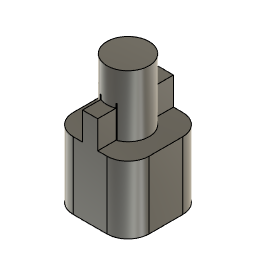
twomes-p1-gateway-button (Autodesk Fusion 360 design; units mm, degrees)
Autodesk Fusion 360 part; units mm, degrees
sketch "Sketch1" plane through (0, 0, 0) normal (0, 1, 0) x (1, 0, 0) in component "RectangleBaseCap"
  line L0 (8.6959, 0, -1.1385) -> (17.6959, 0, -1.1385)
  line L1 (17.6959, 0, -1.1385) -> (17.6959, 0, 7.8615)
  line L2 (17.6959, 0, 7.8615) -> (8.6959, 0, 7.8615)
  line L3 (8.6959, 0, 7.8615) -> (8.6959, 0, -1.1385)
  dimension "d21" = 9
  dimension "d22" = 9
extrude "Extrude1" add sketch "Sketch1" against normal blind 7 contours L0 L1 L2 L3 in plane through (0, 0, 0) normal (0, 0, -1) in component "RectangleBaseCap"
sketch "Sketch2" plane through (0, 0, 7) normal (0, 0, 1) x (-1, 0, 0) in component "RectangleBaseCap"
  line L0 (-8.6959, -7.8615) -> (-8.6959, 1.1385)
  line L1 (-8.6959, 1.1385) -> (-17.6959, 1.1385)
  line L2 (-17.6959, 1.1385) -> (-17.6959, -7.8615)
  line L3 (-17.6959, -7.8615) -> (-8.6959, -7.8615)
  circle A0 centre (-13.1959, -3.3615) radius 2.5
  dimension "d25" = 5
  measures "d25" diameter of A0
extrude "Extrude2" add sketch "Sketch2" along normal blind 5 contours A0 in component "RectangleBaseCap"
move_body "Move1" [no effect]
extrude "Extrude3" add 1 faces at (11.6959, 1.8615, 0) along direction (0, 0, -1) blind 4 in component "RectangleBaseCap"
sketch "Sketch3" plane through (0, 0, -4) normal (0, 0, -1) x (1, 0, 0) in component "RectangleBaseCap"
  line L0 (8.6959, 1.1385) -> (8.6959, -7.8615)
  line L1 (8.6959, -7.8615) -> (17.6959, -7.8615)
  line L2 (17.6959, -7.8615) -> (17.6959, 1.1385)
  line L3 (17.6959, 1.1385) -> (8.6959, 1.1385)
  line L4 (9.6959, -6.8615) -> (16.6959, -6.8615)
  line L5 (16.6959, -6.8615) -> (16.6959, 0.1385)
  line L6 (16.6959, 0.1385) -> (9.6959, 0.1385)
  line L7 (9.6959, 0.1385) -> (9.6959, -6.8615)
  line L8 (8.6959, -3.3615) -> (9.6959, -3.3615) construction
  line L9 (13.1959, -7.8615) -> (13.1959, -6.8615) construction
  dimension "d30" = 7
  dimension "d31" = 7
  constraint horizontal L4
  constraint vertical L5
  constraint horizontal L6
  constraint vertical L7
  constraint midpoint L0 L8.start
  constraint midpoint L7 L8.end
  constraint perpendicular L0 L8
  constraint midpoint L1 L9.start
  constraint midpoint L4 L9.end
  constraint perpendicular L1 L9
  measures "d30" distance of L4.start L6.end
  measures "d31" distance of L5 L7
extrude "Extrude4" cut sketch "Sketch3" against normal blind 4 contours L4 L5 L6 L7 in component "RectangleBaseCap"
sketch "Sketch3 (2)" plane through (0, 0, 7) normal (0, 0, 1) x (-1, 0, 0)
  circle A0 centre (-13.1959, -3.3615) radius 2.5
  line L0 (-8.6959, -7.8615) -> (-8.6959, 1.1385)
  line L1 (-8.6959, 1.1385) -> (-17.6959, 1.1385)
  line L2 (-17.6959, 1.1385) -> (-17.6959, -7.8615)
  line L3 (-17.6959, -7.8615) -> (-8.6959, -7.8615)
  line L4 (-13.1959, -7.8615) -> (-13.1959, 1.1385) construction
  line L5 (-12.1959, 1.1385) -> (-14.1959, 1.1385)
  line L6 (-14.1959, 1.1385) -> (-14.1959, -7.8615)
  line L7 (-14.1959, -7.8615) -> (-12.1959, -7.8615)
  line L8 (-12.1959, -7.8615) -> (-12.1959, 1.1385)
  dimension "d37" = 1
  dimension "d38" = 1
  constraint midpoint L3 L4.start
  constraint midpoint L1 L4.end
  constraint horizontal L5
  constraint vertical L6
  constraint horizontal L7
  constraint vertical L8
  constraint coincident L3 L6.end
  constraint coincident L1 L5.start
  measures "d37" distance of L4 L8
  measures "d38" distance of L4 L6
extrude "Extrude5" add sketch "Sketch3 (2)" along normal blind 3 contours A0 L1 L5 L6 L8 | A0 L3 L6 L7 L8 in component "RectangleBaseCap"
fillet "Fillet1" radius 2.5 4 edges at (8.6959, 7.8615, 1.5) (8.6959, -1.1385, 1.5) (17.6959, -1.1385, 1.5) (17.6959, 7.8615, 1.5) in component "RectangleBaseCap"
extrude "Extrude6" cut 2 faces at (9.3625, 3.3615, 7) (17.0292, 3.3615, 7) along direction (0, 0, -1) blind 0.5 in component "RectangleBaseCap"
extrude "Extrude7" cut 2 faces at (13.1959, 7.1948, 10) (13.1959, -0.4719, 10) along direction (0, 0, -1) blind 0.5 in component "RectangleBaseCap"
extrude "Extrude8" add 1 faces at (13.6857, 2.2646, 12) along direction (0, 0, 1) blind 0.5 in component "RectangleBaseCap"
extrude "Extrude9" cut 2 faces at (17.0292, 3.3615, 6.5) (9.3625, 3.3615, 6.5) along direction (0, 0, -1) blind 1.8 in component "RectangleBaseCap"
extrude "Extrude10" cut 2 faces at (13.1959, -0.4719, 9.5) (13.1959, 7.1948, 9.5) along direction (0, 0, -1) blind 1.5 in component "RectangleBaseCap"
extrude "Extrude11" cut 1 faces at (9.3625, 4.0281, -4) along direction (0, 0, 1) blind 0.2 in component "RectangleBaseCap"
extrude "Extrude12" cut 2 faces at (14.1959, 6.389, 5.8) (14.1959, -0.4023, 5.8) along direction (-1, 0, 0) blind 0.1 in component "RectangleBaseCap"
extrude "Extrude13" cut 2 faces at (12.1959, 7.1252, 6.9) (12.1959, -0.4023, 6.5667) along direction (1, 0, 0) blind 0.1 in component "RectangleBaseCap"
extrude "Extrude14" cut 1 faces at (13.6857, 2.2646, 12.5) along direction (0, 0, -1) blind 1 in component "RectangleBaseCap"
extrude "Extrude15" cut 2 faces at (13.1345, 7.1925, 8) (13.1345, -0.4696, 8) along direction (0, 0, -1) blind 0.5 in component "RectangleBaseCap"
extrude "Extrude16" cut 2 faces at (17.0292, 3.3615, 4.7) (9.3625, 3.3615, 4.7) along direction (0, 0, -1) blind 0.5 in component "RectangleBaseCap"
component "RectangleBaseCap" placed x (1, 0, 0) y (0, 1, 0) z (0, 0, 1) at (0, 0, 0)
equation "CapWidth = 9 mm"
equation "CapHeight = 7 mm"
equation "topDiameter = 5 mm"
equation "topHeight = 5 mm"
equation "buttonWidth = 7 mm"
equation "buttonHeight = 4 mm"
equation "d21 = CapWidth"
equation "d22 = CapWidth"
equation "d23 = CapHeight"
equation "d25 = topDiameter"
equation "d26 = topHeight"
equation "d28 = buttonHeight"
equation "d30 = buttonWidth"
equation "d31 = buttonWidth"
equation "d34 = -buttonHeight"
